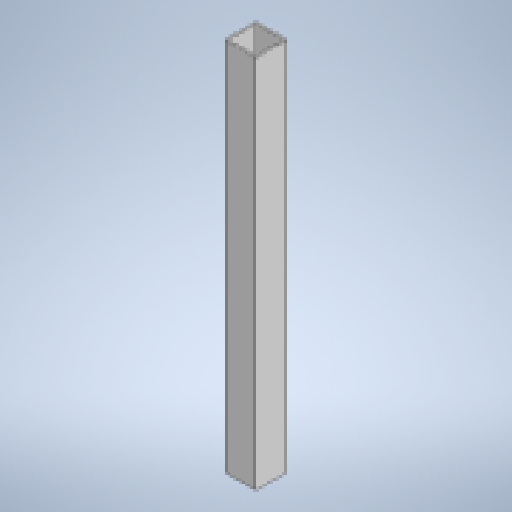
# Autodesk Inventor part: Steel_Tube
Saved by Autodesk Inventor 2023 (Build 270158000, 158)
## iProperties
Created: 2022-04-30
Part Number: Steel_Tube
Material: Generic
Document SubType Name: Modeling
Designer: plebbb
Density: 1 g/cm^3
Appearance: Default
Author: plebbb
Autodesk Inventor part; units mm, degrees
ref_plane "YZ Plane" through (0, 0, 0) normal (1, 0, 0) x (0, 1, 0)
ref_plane "XZ Plane" through (0, 0, 0) normal (0, 1, 0) x (-1, 0, 0)
ref_plane "XY Plane" through (0, 0, 0) normal (0, 0, 1) x (1, 0, 0)
sketch "Sketch1" plane through (0, 0, 0) normal (0, 1, 0) x (-1, 0, 0)
  line L0 (0, 0) -> (25.4, 0)
  line L1 (25.4, 0) -> (25.4, -25.4)
  line L2 (25.4, -25.4) -> (0, -25.4)
  line L3 (0, -25.4) -> (0, 0)
  line L4 (23.8125, -1.5875) -> (1.5875, -1.5875)
  line L5 (1.5875, -1.5875) -> (1.5875, -23.8125)
  line L6 (1.5875, -23.8125) -> (23.8125, -23.8125)
  line L7 (23.8125, -23.8125) -> (23.8125, -1.5875)
  dimension "d0" = 25.4
  dimension "d1" = 1.5875
  dimension "d2" = 1.5875
  dimension "d3" = 1.5875
  constraints: 16 end point, 4 parallel, 4 perpendicular, 2 horizontal, 1 coincident
  measures "d0" distance of L0.end L1.end
  measures "d1" distance between parallel lines of L1 L7
  measures "d2" distance between parallel lines of L2 L6
  measures "d3" distance between parallel lines of L0 L4
extrude "Extrusion1" add sketch "Sketch1" along normal blind 900
body "Solid1"
